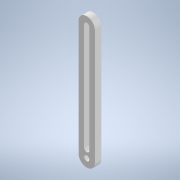
# Autodesk Inventor part: holder
Saved by Autodesk Inventor 2020 (Build 240168000, 168)
## iProperties
Created: 2022-10-15
Part Number: holder
Material: Типовые
Document SubType Name: Modeling
Designer: akapu
Density: 1 g/cm^3
Appearance: По умолчанию
Author: akapu
Autodesk Inventor part; units mm, degrees
ref_plane "YZ Plane" through (0, 0, 0) normal (1, 0, 0) x (0, 1, 0)
ref_plane "XZ Plane" through (0, 0, 0) normal (0, 1, 0) x (-1, 0, 0)
ref_plane "XY Plane" through (0, 0, 0) normal (0, 0, 1) x (1, 0, 0)
sketch "Эскиз1" plane through (0, 0, 0) normal (0, 0, 1) x (1, 0, 0)
  arc A0 (5, 35) -> (-5, 35) centre (0, 35) ccw projected
  line L0 (-5, 35) -> (-5, -35) projected
  arc A1 (-5, -35) -> (5, -35) centre (0, -35) ccw projected
  line L1 (5, -35) -> (5, 35) projected
  arc A2 (-1.6, -30.2629) -> (1.6, -30.2629) centre (0, -30.2629) ccw projected
  line L2 (-1.6, -30.2629) -> (-1.6, 35) projected
  arc A3 (1.6, 35) -> (-1.6, 35) centre (0, 35) ccw projected
  line L3 (1.6, 35) -> (1.6, -30.2629) projected
  circle A4 centre (0, -35) radius 1.6 projected
  point P0 (0, 0)
extrude "Выдавливание1" add sketch "Эскиз1" along normal blind 4
